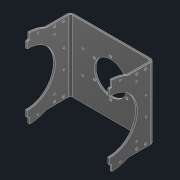
# Autodesk Inventor part: steelplate1
Saved by Autodesk Inventor 2022 (Build 260153000, 153)
## iProperties
Created: 2021-07-14
Part Number: steelplate1
Material: 鋼、炭素鋼
Document SubType Name: Sheet Metal
Designer: yuta0
Density: 7.85 g/cm^3
Sheet Metal Rule: Default_mm
Appearance: 滑らか - 黒
Mass: 644.861 g
Surface Area: 559.257 cm^2
Volume: 82.1479 cm^3
購入先: Meviy
在庫数: 0.0
Author: yuta0
Autodesk Inventor part; units mm, degrees
ref_plane "YZ Plane" through (0, 0, 0) normal (1, 0, 0) x (0, 1, 0)
ref_plane "XZ Plane" through (0, 0, 0) normal (0, 1, 0) x (-1, 0, 0)
ref_plane "XY Plane" through (0, 0, 0) normal (0, 0, 1) x (1, 0, 0)
sketch "スケッチ1" plane through (0, 0, 0) normal (0, 0, 1) x (1, 0, 0)
  line L0 (-71.7, -67.5) -> (71.7, -67.5)
  line L1 (71.7, -67.5) -> (71.7, 67.5)
  line L2 (71.7, 67.5) -> (-71.7, 67.5)
  line L3 (-71.7, 67.5) -> (-71.7, -67.5)
  line L4 (-71.7, -67.5) -> (71.7, 67.5) construction
  line L5 (71.7, -67.5) -> (-71.7, 67.5) construction
  point P0 (0, 0)
  dimension "d1" = 135
  dimension "d2" = 143.4
  measures "d1" distance of L2.end L0.start
  measures "d2" distance of L1.end L2.end
extrude "プレート1" add sketch "スケッチ1" along normal blind 3.2
sketch "スケッチ2" plane through (-68.5, -67.5, 0) normal (-1, 0, 0) x (0, -1, 0)
  line L0 (-135, 0) -> (0, 0)
  line L1 (0, 0) -> (0, 142)
  line L2 (0, 142) -> (-135, 142)
  line L3 (-135, 142) -> (-135, 0)
  constraints: 6 end point, 1 horizontal, 1 perpendicular, 1 vertical
edge flange "フランジ1" height 142 angle 90 thickness 3.2 bend radius 3.2 thickness toward (-1, 0, 0) relief tear relief width 3.2 relief depth 1.6 corner gap 3.2 corner form 0 edges at (-71.7, 0, 3.2) (71.7, 0, 3.2) wall of the first edge with corners at (-68.5, 67.5, 0) (-68.5, -67.5, 0) (-68.5, -67.5, 142) (-68.5, 67.5, 142)
bend "曲げ1"
corner "コーナー1"
sketch "スケッチ4" plane through (71.7, -67.5, 6.4) normal (1, 0, 0) x (0, 0, -1)
  circle A0 centre (-68.1, 67.5) radius 45.5
  line L0 (-135.6, 0) -> (-135.6, 135) projected
  line L1 (-135.6, 135) -> (0, 135) projected
  point P0 (6.4, 67.5)
  dimension "d17" = 91
  dimension "d54" = 67.5
  dimension "d55" = 67.5
  constraints: 1 centre point
  measures "d17" diameter of A0
  measures "d54" distance from line of L0 A0.centre
  measures "d55" distance from line of L1 A0.centre
extrude "押し出し2" cut sketch "スケッチ4" against normal through all
sketch "スケッチ5" plane through (71.7, -67.5, 6.4) normal (1, 0, 0) x (0, 0, -1)
  circle A0 centre (-68.1, 67.5) radius 62.5
  circle A1 centre (-68.1, 67.5) radius 45.5 projected
  point P0 (6.4, 67.5)
  point P1 (-128.4704, 51.3238)
  point P2 (-112.2942, 23.3058)
  point P3 (-84.2762, 7.1296)
  point P4 (-51.9238, 7.1296)
  point P5 (-23.9058, 23.3058)
  point P6 (-7.7296, 51.3238)
  point P7 (-7.7296, 83.6762)
  point P8 (-23.9058, 111.6942)
  point P9 (-51.9238, 127.8704)
  point P10 (-84.2762, 127.8704)
  point P11 (-112.2942, 111.6942)
  point P12 (-128.4704, 83.6762)
  dimension "d20" = 125
  dimension "d23" = 360
  dimension "d71" = 0
  constraints: 1 coincident, 16 other
  measures "d71" horizontal distance of point (-128.47, 83.676) point (-128.47, 51.324)
hole "穴1" at (71.7, 16.1762, 134.8704) at (71.7, 44.1942, 118.6942) at (71.7, 60.3704, 90.6762) at (71.7, 60.3704, 58.3238) at (71.7, 44.1942, 30.3058) at (71.7, -16.1762, 14.1296) at (71.7, -44.1942, 30.3058) at (71.7, -60.3704, 58.3238) at (71.7, -60.3704, 90.6762) at (71.7, -44.1942, 118.6942) at (71.7, -16.1762, 134.8704) at (71.7, 16.1762, 14.1296) direction (-1, 0, 0) diameter 3.242 end through all thread size "M4x0.7" class "6H" standard "ANSI Metric M Profile"
sketch "スケッチ6" plane through (0, 0, 3.2) normal (0, 0, 1) x (1, 0, 0)
  circle A0 centre (0, 0) radius 32
  point P0 (0, 32)
  point P1 (-27.7128, 16)
  point P2 (-27.7128, -16)
  point P3 (0, -32)
  point P4 (27.7128, -16)
  point P5 (27.7128, 16)
  dimension "d32" = 64
  dimension "d35" = 360
  constraints: 1 coincident, 1 vertical alignment, 9 other
hole "穴2" at (0, 32, 3.2) at (-27.7128, 16, 3.2) at (-27.7128, -16, 3.2) at (0, -32, 3.2) at (27.7128, -16, 3.2) at (27.7128, 16, 3.2) direction (0, 0, -1) diameter 4.3 end through all clearance for "Flat Head Machine Screw" size "M4" standard "Ansi Metric M Profile"
sketch "スケッチ7" plane through (0, 0, 3.2) normal (0, 0, 1) x (1, 0, 0)
  circle A0 centre (0, 0) radius 28
  dimension "d44" = 56
  constraints: 1 centre point, 1 coincident
  measures "d44" diameter of A0
extrude "押し出し3" cut sketch "スケッチ7" against normal blind 10
sketch "スケッチ8" plane through (71.7, -67.5, 6.4) normal (1, 0, 0) x (0, 0, -1)
  line L0 (-135.6, 0) -> (-68.1, 0)
  line L1 (-68.1, 0) -> (-68.1, 135)
  line L2 (-68.1, 135) -> (-135.6, 135)
  line L3 (-135.6, 135) -> (-135.6, 0)
  circle A0 centre (-68.1, 67.5) radius 45.5 projected
  line L4 (0, 0) -> (-135.6, 0) projected
  line L5 (-135.6, 135) -> (0, 135) projected
  circle A1 centre (-68.1, 67.5) radius 67.5
  line L6 (-66.1, 0.0296) -> (-66.1, 11.0296)
  line L7 (-66.1, 11.0296) -> (-70.1, 11.0296)
  line L8 (-70.1, 11.0296) -> (-70.1, 22.044)
  line L9 (-164, 67.5) -> (34.8, 67.5) projected
  line L10 (-66.1, 134.9704) -> (-66.1, 123.9704)
  line L11 (-66.1, 123.9704) -> (-70.1, 123.9704)
  line L12 (-70.1, 123.9704) -> (-70.1, 112.956)
  point P0 (6.4, 67.5)
  point P1 (-70.1, 112.956)
  point P2 (-66.1, 134.9704)
  point P3 (-68.1, 135)
  dimension "d56" = 0
  dimension "d150" = 2
  dimension "d151" = 2
  dimension "d152" = 11
  constraints: 21 end point, 4 symmetric about line, 2 parallel, 2 perpendicular, 2 point on circle, 2 point on line, 1 centre point, 1 coincident, 1 horizontal, 2 other
  measures "d56" distance from line of point (-68.1, 67.5) L1
  measures "d150" distance between parallel lines of L1 L8
  measures "d151" distance between parallel lines of L1 L6
  measures "d152" distance of L6.start L6.end
extrude "押し出し4" cut sketch "スケッチ8" against normal through all contours L3 A1 L0 | A1 L9 A0 L8 L7 L1 | L1 L7 L6 A1 | L3 L2 A1 | A1 L1 L11 L12 A0 L9 | A1 L10 L11 L1
sketch "スケッチ15" plane through (0, 0, 3.2) normal (0, 0, 1) x (1, 0, 0)
  line L0 (-47.45, -20) -> (47.45, -20)
  line L1 (47.45, -20) -> (47.45, 20)
  line L2 (47.45, 20) -> (-47.45, 20)
  line L3 (-47.45, 20) -> (-47.45, -20)
  line L4 (-47.45, -20) -> (47.45, 20) construction
  line L5 (47.45, -20) -> (-47.45, 20) construction
  point P0 (0, 0)
  dimension "d122" = 94.9
  dimension "d123" = 40
  constraints: 12 end point, 2 midpoint, 2 parallel, 1 horizontal, 1 perpendicular
  measures "d122" distance of L1.end L2.end
  measures "d123" distance of L0.end L1.end
hole "穴6" at (-47.45, 20, 3.2) at (47.45, 20, 3.2) at (47.45, -20, 3.2) at (-47.45, -20, 3.2) direction (0, 0, -1) diameter 3.242 end through all thread size "M4x0.7" class "6H" standard "ANSI Metric M Profile"
sketch "スケッチ17" plane through (0, 0, 0) normal (1, 0, 0) x (0, 1, 0)
  line L0 (-67.5, 6.4) -> (-67.5, 0) projected
  line L1 (-67.5, 6.4) -> (-67.5, 74.5) projected
  line L2 (-67.5, 0) -> (-60.5, 0)
  line L3 (-60.5, 0) -> (-60.5, 44.5667)
  line L4 (-60.5, 44.5667) -> (-67.5, 44.5667)
  line L5 (-67.5, 44.5667) -> (-67.5, 0)
  arc A0 (-45.456, 76.5) -> (45.456, 76.5) centre (0, 74.5) ccw projected
  circle A1 centre (0, 74.5) radius 67.5
  point P0 (0, 0)
  point P1 (-67.5, 75.5)
  point P2 (45.5, 75.5)
  point P3 (-45.5, 75.5)
  point P4 (-67.5, 74.5)
  dimension "d144" = 135
  dimension "d143" = 7
  constraints: 8 end point, 2 parallel, 1 coincident, 1 horizontal, 1 perpendicular, 3 other
  measures "d143" distance of L3.end L4.end
extrude "押し出し9" cut sketch "スケッチ17" along normal through all both and the other way through all contours L1 L4 L3 L2 L0 | L1 A1 L4
mirror "ミラー2" about plane through (0, 0, 0) normal (0, 1, 0) of "押し出し9"
sketch "スケッチ9" plane through (71.7, -67.5, 6.4) normal (1, 0, 0) x (0, 0, -1)
  line L0 (0, 0) -> (0, 135) projected
  line L1 (0, 0) -> (-69.1, 0) projected
  arc A0 (-70.1, 22.044) -> (-70.1, 112.956) centre (-68.1, 67.5) ccw projected
  circle A1 centre (-68.1, 67.5) radius 67.5
  line L2 (-69.1, 135) -> (0, 135) projected
  line L3 (0, 128) -> (-38.1667, 128) projected
  point P0 (6.4, 67.5)
  point P1 (-23.6, 123)
  point P2 (-64.4, 0)
  point P3 (-69.1, 113)
  point P4 (-39.1667, 128)
  point P5 (-8.6, 123)
  dimension "d60" = 135
  dimension "d147" = 5
  dimension "d154" = 23.6
  dimension "d155" = 15
  dimension "d156" = 5
  constraints: 1 coincident, 2 other
  measures "d147" distance from line of L3 point (-23.6, 123)
  measures "d154" distance from line of L0 point (-23.6, 123)
  measures "d155" distance of point (-23.6, 123) point (-8.6, 123)
  measures "d156" distance from line of L3 point (-8.6, 123)
hole "穴3" at (71.7, 55.5, 30) at (71.7, 55.5, 15) direction (-1, 0, 0) diameter 4.3 end through all clearance for "Flat Head Machine Screw" size "M4" standard "Ansi Metric M Profile"
fillet "コーナーR9" radius 10 4 edges at (70.1, 60.5, 44.5667) (-70.1, 60.5, 44.5667) (70.1, -60.5, 44.5667) (-70.1, -60.5, 44.5667)
mirror "ミラー3" about plane through (0, 0, 0) normal (0, 1, 0) of "穴3"
fillet "コーナーR10" radius 1 8 edges at (-70.1, 56.4704, 72.5) (-70.1, 56.4704, 76.5) (-70.1, -56.4704, 76.5) (-70.1, -56.4704, 72.5) (70.1, 56.4704, 76.5) (70.1, 56.4704, 72.5) (70.1, -56.4704, 72.5) (70.1, -56.4704, 76.5)
equation "\"d30\" = Thickness"
equation "\"d42\" = Thickness"
equation "\"d129\" = Thickness"
equation "\"d68\" = Thickness"
equation "\"d3\" = Thickness"
equation "\"d4\" = BendReliefWidth"
equation "\"d5\" = BendReliefDepth"
equation "\"d6\" = MinimumRemnant"
equation "\"d7\" = TransitionRadius"
equation "\"d10\" = BendRadius"
equation "\"d11\" = CornerReliefSize"
equation "\"d12\" = GapSize"
equation "\"d13\" = JacobiRadiusSize"
equation "\"BendRadius\" = Thickness"
equation "\"BendReliefWidth\" = Thickness"
equation "\"BendReliefDepth\" = 0.5 * Thickness"
equation "\"CornerReliefSize\" = 4 * Thickness"
equation "\"MinimumRemnant\" = 2 * Thickness"
equation "\"TransitionRadius\" = BendRadius"
equation "\"JacobiRadiusSize\" = BendRadius"
equation "\"GapSize\" = Thickness"
equation "\"Thickness\" = 3.2"
